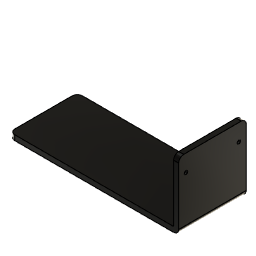
solar tracker v4 (Autodesk Fusion 360 archive; units mm, degrees)
design "PEZZO2"
Autodesk Fusion 360 part; units mm, degrees
sketch "Schizzo1" plane through (0, 0, 0) normal (0, 1, 0) x (1, 0, 0)
  line L0 (-155, 0) -> (-55, 0)
  line L1 (-55, 0) -> (-55, -40)
  line L2 (-155, -3) -> (-58, -3)
  line L3 (-58, -3) -> (-58, -40)
  line L4 (-155, 0) -> (-155, -3)
  line L5 (-55, -40) -> (-58, -40)
  dimension "d1" = 100
  dimension "d2" = 40
  dimension "d3" = 3
  constraint horizontal L0
  constraint perpendicular L0 L1
  measures "d1" distance of L0.start L0.end
  measures "d2" distance of L0.end L1.end
extrude "Estrusione1" add sketch "Schizzo1" along normal mid plane 40 makes body 1
fillet "Raccordo1" radius 3 4 edges at (-56.5, -20, 40) (-56.5, 20, 40) (-155, -20, 1.5) (-155, 20, 1.5) on bodies 1
fillet "Raccordo2" radius 3 1 edges at (-55, 0, 0) on bodies 1
fillet "Raccordo2" radius 0.5 1 edges at (-58, 0, 3) on bodies 1
sketch "Schizzo2" plane through (-55, 0, 0) normal (1, 0, 0) x (0, 1, 0)
  line L0 (-20, 3) -> (20, 3)
  line L1 (20, 3) -> (20, 37)
  arc A0 (20, 37) -> (17, 40) centre (17, 37) ccw
  line L2 (17, 40) -> (-17, 40)
  arc A1 (-17, 40) -> (-20, 37) centre (-17, 37) ccw
  line L3 (-20, 37) -> (-20, 3)
  circle A2 centre (-15.65, 30) radius 1
  circle A3 centre (15.65, 30) radius 1
  line L4 (-15.65, 30) -> (15.65, 30) construction
  line L5 (0, 30) -> (0, 40) construction
  dimension "d12" = 2
  dimension "d13" = 2
  dimension "d14" = 10
  dimension "d15" = 31.3
  constraint coincident A2.centre L4.start
  constraint horizontal L4
  constraint coincident A3.centre L4.end
  constraint midpoint L4 L5.start
  constraint midpoint L2 L5.end
  constraint vertical L5
  measures "d12" diameter of A2
  measures "d13" diameter of A3
  measures "d14" distance of L2 L4
  measures "d15" distance of A2.centre A3.centre
extrude "Estrusione2" cut sketch "Schizzo2" against normal through all contours A2 | A3 bodies 1
copy_body "Corpo->Comp1" bodies 1 removing the originals makes body 2 in component "Component"
component "Component" placed x (1, 0, 0) y (0, 1, 0) z (0, 0, 1) at (0, 0, 0)
